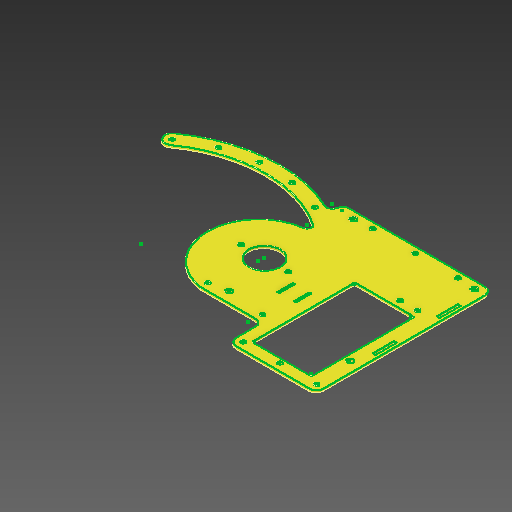
# Autodesk Inventor part: wstepna_geometria_wersja_2
Saved by Autodesk Inventor 2022 (Build 260153000, 153)
## iProperties
Created: 2022-02-09
Part Number: wstepna_geometria_wersja_2
Material: Aluminum 6061
Document SubType Name: Modeling
Designer: Tomasz Krakowski
Density: 2.7 g/cm^3
Appearance: Kanarkowa
Mass: 59.5222 g
Surface Area: 247.106 cm^2
Volume: 22.0453 cm^3
Author: Tomasz Krakowski
Autodesk Inventor part; units mm, degrees
ref_plane "YZ Plane" through (0, 0, 0) normal (1, 0, 0) x (0, 1, 0)
ref_plane "XZ Plane" through (0, 0, 0) normal (0, 1, 0) x (-1, 0, 0)
ref_plane "XY Plane" through (0, 0, 0) normal (0, 0, 1) x (1, 0, 0)
sketch "Sketch1" plane through (0, 0, 0) normal (0, 1, 0) x (-1, 0, 0)
  arc A0 (-0.3814, 2.9757) -> (-3, 0) centre (0, 0) ccw
  circle A1 centre (-5, 35) radius 11
  arc A2 (-0.3814, 2.9757) -> (0, 75) centre (-5, 39.0133) ccw
  line L0 (-105, 0) -> (0, 0) construction
  line L1 (-3, 0) -> (-105, 0) construction
  arc A3 (-3, 0) -> (-0.3814, -2.9757) centre (0, 0) ccw
  arc A4 (-1.6619, -2.4976) -> (97.0992, -0.9275) centre (46.5785, 70) ccw
  arc A5 (102.9008, -9.0725) -> (97.0992, -0.9275) centre (100, -5) ccw
  line L2 (0, 0) -> (100, 0) construction
  arc A6 (5.6849, -18.0476) -> (102.9008, -9.0725) centre (46.5785, 70) ccw
  line L3 (0, 75) -> (0, 0) construction
  line L4 (0, 0) -> (0, -15.1769) construction
  line L5 (0, 0) -> (-105, 0) construction
  line L6 (0, 75) -> (-105, 75)
  line L7 (-105, 75) -> (-105, -25)
  line L8 (0, -21.6754) -> (0, -21)
  line L9 (-4, -25) -> (-105, -25)
  arc A7 (5.6849, -18.0476) -> (0, -21.6754) centre (4, -21.6754) ccw
  arc A8 (-4, -25) -> (0, -21) centre (-4, -21) ccw
  point P0 (-5, -39.0133)
  point P1 (0, -25)
  dimension "d0" = 6
  dimension "d7" = 22
  dimension "d13" = 5
  dimension "d47" = 10
  dimension "d49" = 100
  dimension "d68" = 70
  dimension "d71" = 0
  dimension "d75" = 105
  dimension "d76" = 4
  dimension "d77" = 4
  dimension "d101" = 100
  dimension "d105" = 75
  dimension "d106" = 35
  dimension "d107" = 5
  constraints: 20 end point, 19 point on circle, 9 centre point, 9 tangent, 6 point on line, 5 horizontal, 3 coincident, 2 symmetric about line, 2 vertical, 1 collinear, 1 perpendicular, 1 other
  measures "d0" diameter of A0
  measures "d7" diameter of A1
  measures "d13" horizontal distance of point (0, 0) A2.centre
  measures "d47" diameter of A5
  measures "d49" horizontal distance of point (0, 0) A5.centre
  measures "d68" vertical distance of point (0, 0) A4.centre
  measures "d71" distance between parallel lines of L5 L1
  measures "d75" horizontal distance of point (0, 0) L6.end
  measures "d76" radius of A7
  measures "d77" radius of A8
  measures "d101" distance between parallel lines of L6 L9
  measures "d105" distance from line of L6 point (0, 0)
  measures "d106" vertical distance of point (0, 0) A1.centre
  measures "d107" horizontal distance of point (0, 0) A1.centre
extrude "Extrusion1" add sketch "Sketch1" along normal blind 2
sketch "Szkic5" plane through (0, 2, 0) normal (0, 1, 0) x (1, 0, 0)
  circle A0 centre (12.5, 20) radius 2.1
  circle A1 centre (97.5, 20) radius 2.1
  circle A2 centre (12.5, -67.5) radius 2.1
  circle A3 centre (97.5, -67.5) radius 2.1
  line L0 (12.5, 20) -> (97.5, 20) construction
  line L1 (97.5, -67.5) -> (97.5, 20) construction
  line L2 (12.5, -67.5) -> (97.5, -67.5) construction
  line L3 (0, -75) -> (105, -75) construction
  line L4 (105, -75) -> (105, 25) construction
  line L5 (105, 25) -> (4, 25) construction
  line L6 (0, 21) -> (0, 21.6754) construction
  line L7 (12.5, 20) -> (12.5, -67.5) construction
  point P0 (0, 0)
  dimension "d84" = 7.5
  dimension "d85" = 7.5
  dimension "d88" = 4.2
  dimension "d89" = 85
  dimension "d109" = 87.5
  constraints: 8 end point, 4 centre point, 3 equal radius, 2 horizontal, 1 perpendicular, 1 vertical
  measures "d84" distance between parallel lines of L3 L2
  measures "d85" distance between parallel lines of L4 L1
  measures "d88" diameter of A0
  measures "d89" distance of L2.start L1.start
  measures "d109" distance between parallel lines of L2 L0
extrude "Wyciągnięcie proste4" cut sketch "Szkic5" against normal up to surface (2 mm away)
sketch "Szkic6" plane through (0, 2, 0) normal (0, 1, 0) x (1, 0, 0)
  line L0 (103, -55) -> (100.9, -55)
  line L1 (100.9, -55) -> (100.9, -40)
  line L2 (100.9, -40) -> (103, -40)
  line L3 (103, -40) -> (103, -55)
  line L4 (103, -10) -> (100.9, -10)
  line L5 (100.9, -10) -> (100.9, 5)
  line L6 (100.9, 5) -> (103, 5)
  line L7 (103, 5) -> (103, -10)
  line L8 (100.9, -40) -> (100.9, -10) construction
  line L9 (100.9, -25) -> (105, -25) construction
  line L10 (105, -75) -> (105, 25) construction
  point P0 (0, 0)
  point P1 (105, 25)
  dimension "d92" = 15
  dimension "d94" = 30
  dimension "d127" = 2.1
  dimension "d128" = 2
  constraints: 20 end point, 4 parallel, 3 perpendicular, 2 collinear, 2 horizontal, 1 midpoint, 1 point on line, 2 other
  measures "d92" distance of L4.end L5.end
  measures "d94" distance between parallel lines of L4 L2
  measures "d127" distance of L5.end L6.end
extrude "Wyciągnięcie proste5" cut sketch "Szkic6" against normal up to surface (2 mm away)
sketch "Sketch8" plane through (0, 2, 0) normal (0, 1, 0) x (1, 0, 0)
  circle A0 centre (-11.5, -35) radius 1.6
  circle A1 centre (21.5, -35) radius 1.6
  circle A2 centre (5, -35) radius 11 construction
  line L0 (-11.5, -35) -> (21.5, -35) construction
  point P0 (0, 0)
  dimension "d110" = 33
  dimension "d111" = 3.2
  constraints: 2 centre point, 2 end point, 1 coincident, 1 equal radius, 1 horizontal, 1 midpoint
  measures "d110" distance of L0.start L0.end
  measures "d111" diameter of A0
extrude "Extrusion6" cut sketch "Sketch8" against normal through all
fillet "Fillet1" radius 5 1 edges at (105, 1, -25)
sketch "Sketch9" plane through (0, 2, 0) normal (0, 1, 0) x (1, 0, 0)
  line L0 (0, -75) -> (105, -75) projected
  line L1 (105, -75) -> (105, -98.5)
  line L2 (105, -98.5) -> (43.5, -98.5)
  line L3 (43.5, -98.5) -> (43.5, -75)
  line L4 (43.5, -75) -> (51.5, -75)
  line L5 (51.5, -75) -> (51.5, -90.5)
  line L6 (51.5, -90.5) -> (93.5, -90.5)
  line L7 (93.5, -90.5) -> (93.5, -75)
  line L8 (105, -75) -> (93.5, -75)
  point P0 (0, 0)
  dimension "d116" = 8
  dimension "d117" = 8
  dimension "d118" = 15.5
  dimension "d119" = 42
  dimension "d130" = 51.5
  constraints: 16 end point, 4 perpendicular, 3 point on line, 2 vertical
  measures "d116" distance between parallel lines of L3 L5
  measures "d117" distance between parallel lines of L2 L6
  measures "d118" distance between parallel lines of L6 L0
  measures "d119" distance between parallel lines of L7 L5
  measures "d130" distance from line of point (0, 0) L5
extrude "Extrusion7" add sketch "Sketch9" against normal up to surface (2 mm away) contours L0 L5 L6 L7 L1 L2 L3
sketch "Sketch10" plane through (0, 2, 0) normal (0, 1, 0) x (1, 0, 0)
  line L0 (93.5, -75) -> (51.5, -75) projected
  line L1 (51.5, -75) -> (93.5, -75)
  line L2 (93.5, -75) -> (93.5, -18)
  line L3 (93.5, -18) -> (51.5, -18)
  line L4 (51.5, -18) -> (51.5, -75)
  point P0 (0, 0)
  dimension "d123" = 57
  constraints: 8 end point, 2 parallel, 1 horizontal, 1 perpendicular
  measures "d123" distance between parallel lines of L0 L3
extrude "Extrusion8" cut sketch "Sketch10" against normal up to surface (2 mm away)
fillet "Fillet2" radius 5 3 edges at (105, 1, 98.5) (43.5, 1, 98.5) (43.5, 1, 75)
fillet "Fillet3" radius 1 4 edges at (51.5, 1, 18) (93.5, 1, 18) (93.5, 1, 90.5) (51.5, 1, 90.5)
sketch "Sketch11" plane through (0, 2, 0) normal (0, 1, 0) x (1, 0, 0)
  line L0 (78.5, -13) -> (90.5, -13) construction
  line L1 (52.5, -18) -> (92.5, -18) construction
  line L2 (93.5, -19) -> (93.5, -89.5) construction
  point P0 (0, 0)
  dimension "d131" = 5
  dimension "d132" = 3
  dimension "d133" = 12
  constraints: 2 end point, 1 horizontal
  measures "d131" distance between parallel lines of L0 L1
  measures "d132" distance from line of L0.end L2
  measures "d133" distance of L0.end L0.start
hole "Hole1" at (78.5, 2, 13) at (90.5, 2, 13) direction (0, -1, 0) diameter 3.2 end through all
sketch "Sketch12" plane through (0, 2, 0) normal (0, 1, 0) x (1, 0, 0)
  arc A0 (1.6619, 2.4976) -> (-97.0992, 0.9275) centre (-46.5785, -70) ccw construction
  arc A1 (-102.9008, 9.0725) -> (-97.0992, 0.9275) centre (-100, 5) ccw construction
  arc A2 (13.245, 0) -> (-100, 5) centre (-46.5785, -70) ccw construction
  line L0 (-46.5785, -70) -> (-100, 5) construction
  arc A3 (100, -98.5) -> (105, -93.5) centre (100, -93.5) ccw construction
  arc A4 (43.5, -93.5) -> (48.5, -98.5) centre (48.5, -93.5) ccw construction
  line L1 (25, 21) -> (85, 21) construction
  line L2 (100, 25) -> (4, 25) construction
  line L3 (48.5, -93.5) -> (100, -93.5) construction
  line L4 (0, -70) -> (38.5, -70) construction
  line L5 (0, -75) -> (38.5, -75) construction
  line L6 (38.5, -70) -> (38.5, -75) construction
  arc A5 (43.5, -80) -> (38.5, -75) centre (38.5, -80) ccw construction
  arc A6 (0.3814, -2.9757) -> (0, -75) centre (5, -39.0133) ccw construction
  line L7 (0, -75) -> (0, -70) construction
  circle A7 centre (12.5, 20) radius 2.1 construction
  circle A8 centre (97.5, 20) radius 2.1 construction
  line L8 (0, 0) -> (13.245, 0) construction
  point P0 (-78.7683, 16.2709)
  point P1 (-55.3429, 21.6626)
  point P2 (-31.3202, 20.8077)
  point P3 (-8.3374, 13.7643)
  point P4 (55, 21)
  point P5 (74.25, -93.5)
  dimension "d143" = 60
  dimension "d145" = 60
  dimension "d146" = 4
  dimension "d147" = 5
  dimension "d148" = 12.5
  dimension "d149" = 12.5
  constraints: 14 end point, 8 coincident, 4 horizontal, 2 midpoint, 2 perpendicular, 2 point on circle, 1 centre point, 5 other
  measures "d145" distance of L1.start L1.end
  measures "d146" distance between parallel lines of L2 L1
  measures "d147" distance between parallel lines of L5 L4
  measures "d148" horizontal distance of point (25, 21) A7.centre
  measures "d149" horizontal distance of A8.centre L1.end
hole "Hole2" at (-100, 2, -5) at (-78.7683, 2, -16.2709) at (-55.3429, 2, -21.6626) at (-31.3202, 2, -20.8077) at (-8.3374, 2, -13.7643) at (48.5, 2, 93.5) at (100, 2, 93.5) at (25, 2, -21) at (85, 2, -21) at (55, 2, -21) at (74.25, 2, 93.5) at (0, 2, 70) at (38.5, 2, 70) direction (0, -1, 0) diameter 3.2 end through all
sketch "Sketch15" plane through (0, 2, 0) normal (0, 1, 0) x (1, 0, 0)
  line L0 (30, -40) -> (31.5, -40)
  line L1 (31.5, -40) -> (31.5, -51)
  line L2 (31.5, -51) -> (30, -51)
  line L3 (30, -51) -> (30, -40)
  line L4 (41.5, -40) -> (43, -40)
  line L5 (43, -40) -> (43, -51)
  line L6 (43, -51) -> (41.5, -51)
  line L7 (41.5, -51) -> (41.5, -40)
  point P0 (0, 0)
  dimension "d157" = 11
  dimension "d158" = 10
  dimension "d159" = 1.5
  dimension "d160" = 40
  dimension "d161" = 30
  constraints: 16 end point, 4 parallel, 2 horizontal, 2 perpendicular, 2 point on line, 1 collinear
  measures "d157" distance from line of L6.end L4
  measures "d158" distance between parallel lines of L7 L1
  measures "d159" distance of L0.start L0.end
  measures "d160" vertical distance of point (0, 0) L0.start
  measures "d161" distance from line of point (0, 0) L3
extrude "Extrusion9" cut sketch "Sketch15" against normal through all
sketch "Sketch16" plane through (0, 2, 0) normal (0, 1, 0) x (1, 0, 0)
  line L0 (43, -40) -> (43, -51) projected
  line L1 (43, -51) -> (41.5, -51) projected
  line L2 (41.5, -51) -> (41.5, -40) projected
  line L3 (41.5, -40) -> (43, -40) projected
  line L4 (31.5, -40) -> (31.5, -51) projected
  line L5 (31.5, -51) -> (30, -51) projected
  line L6 (30, -51) -> (30, -40) projected
  line L7 (30, -40) -> (31.5, -40) projected
  circle A0 centre (0, -70) radius 1.6 projected
  circle A1 centre (55, 21) radius 1.6 projected
  circle A2 centre (25, 21) radius 1.6 projected
  circle A3 centre (48.5, -93.5) radius 1.6 projected
  circle A4 centre (-31.3202, 20.8077) radius 1.6 projected
  circle A5 centre (-78.7683, 16.2709) radius 1.6 projected
  circle A6 centre (-100, 5) radius 1.6 projected
  circle A7 centre (-55.3429, 21.6626) radius 1.6 projected
  circle A8 centre (-8.3374, 13.7643) radius 1.6 projected
  circle A9 centre (100, -93.5) radius 1.6 projected
  circle A10 centre (85, 21) radius 1.6 projected
  circle A11 centre (74.25, -93.5) radius 1.6 projected
  circle A12 centre (38.5, -70) radius 1.6 projected
  circle A13 centre (78.5, -13) radius 1.6 projected
  circle A14 centre (90.5, -13) radius 1.6 projected
  arc A15 (43.5, -93.5) -> (48.5, -98.5) centre (48.5, -93.5) ccw projected
  line L8 (48.5, -98.5) -> (100, -98.5) projected
  arc A16 (100, -98.5) -> (105, -93.5) centre (100, -93.5) ccw projected
  line L9 (105, -93.5) -> (105, 20) projected
  arc A17 (105, 20) -> (100, 25) centre (100, 20) ccw projected
  line L10 (100, 25) -> (4, 25) projected
  arc A18 (4, 25) -> (0, 21) centre (4, 21) ccw projected
  line L11 (0, 21) -> (0, 21.6754) projected
  arc A19 (-5.6849, 18.0476) -> (0, 21.6754) centre (-4, 21.6754) ccw projected
  arc A20 (-5.6849, 18.0476) -> (-102.9008, 9.0725) centre (-46.5785, -70) ccw projected
  arc A21 (-102.9008, 9.0725) -> (-97.0992, 0.9275) centre (-100, 5) ccw projected
  arc A22 (1.6619, 2.4976) -> (-97.0992, 0.9275) centre (-46.5785, -70) ccw projected
  arc A23 (0.3814, -2.9757) -> (1.6619, 2.4976) centre (0, 0) ccw projected
  arc A24 (0.3814, -2.9757) -> (0, -75) centre (5, -39.0133) ccw projected
  line L12 (0, -75) -> (38.5, -75) projected
  arc A25 (43.5, -80) -> (38.5, -75) centre (38.5, -80) ccw projected
  line L13 (43.5, -80) -> (43.5, -93.5) projected
  line L14 (93.5, -19) -> (93.5, -89.5) projected
  arc A26 (92.5, -90.5) -> (93.5, -89.5) centre (92.5, -89.5) ccw projected
  line L15 (92.5, -90.5) -> (52.5, -90.5) projected
  arc A27 (51.5, -89.5) -> (52.5, -90.5) centre (52.5, -89.5) ccw projected
  line L16 (51.5, -89.5) -> (51.5, -19) projected
  arc A28 (52.5, -18) -> (51.5, -19) centre (52.5, -19) ccw projected
  line L17 (52.5, -18) -> (92.5, -18) projected
  arc A29 (93.5, -19) -> (92.5, -18) centre (92.5, -19) ccw projected
  circle A30 centre (-11.5, -35) radius 1.6 projected
  circle A31 centre (21.5, -35) radius 1.6 projected
  line L18 (103, -55) -> (100.9, -55) projected
  line L19 (100.9, -55) -> (100.9, -40) projected
  line L20 (100.9, -40) -> (103, -40) projected
  line L21 (103, -40) -> (103, -55) projected
  line L22 (100.9, -10) -> (100.9, 5) projected
  line L23 (100.9, 5) -> (103, 5) projected
  line L24 (103, 5) -> (103, -10) projected
  line L25 (103, -10) -> (100.9, -10) projected
  circle A32 centre (12.5, -67.5) radius 2.1 projected
  circle A33 centre (97.5, -67.5) radius 2.1 projected
  circle A34 centre (97.5, 20) radius 2.1 projected
  circle A35 centre (12.5, 20) radius 2.1 projected
  circle A36 centre (5, -35) radius 11 projected
sketch "Sketch17" plane through (0, 2, 0) normal (0, 1, 0) x (1, 0, 0)
  circle A0 centre (14, 7) radius 7.5
  line L0 (100, 25) -> (4, 25) construction
  line L1 (105, -93.5) -> (105, 20) construction
  circle A1 centre (32, 7) radius 7.5
  circle A2 centre (50, 7) radius 7.5
  circle A3 centre (68, 7) radius 7.5
  circle A4 centre (86, 7) radius 7.5
  line L2 (5, -35) -> (5, -13) construction
  circle A5 centre (5, -13) radius 7.5
  circle A6 centre (-14.0526, -24) radius 7.5
  circle A7 centre (-14.0526, -46) radius 7.5
  circle A8 centre (5, -57) radius 7.5
  circle A9 centre (23, -9) radius 7.5
  circle A10 centre (41, -9) radius 7.5
  point P0 (0, 0)
  dimension "d164" = 15
  dimension "d165" = 14
  dimension "d166" = 7
  dimension "d169" = 18
  dimension "d174" = 22
  dimension "d177" = 180
  dimension "d179" = 16
  dimension "d180" = 9
  dimension "d183" = 18
  constraints: 11 centre point, 3 coincident, 2 end point, 2 equal radius, 2 horizontal, 1 vertical, 19 other
  measures "d164" diameter of A0
  measures "d165" horizontal distance of point (0, 0) A0.centre
  measures "d166" vertical distance of point (0, 0) A0.centre
  measures "d169" distance of A0.centre A1.centre
  measures "d174" distance of L2.start L2.end
  measures "d179" vertical distance of A0.centre A9.centre
  measures "d180" horizontal distance of A0.centre A9.centre
  measures "d183" distance of A9.centre A10.centre
body "Solid1"
